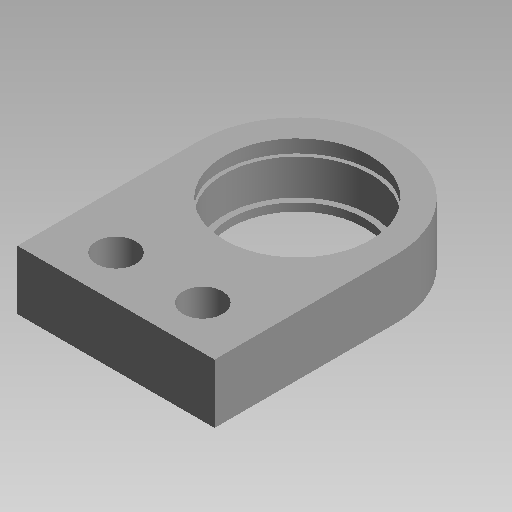
# Autodesk Inventor part: SBGSMA6904ZZ-35_h
Saved by Autodesk Inventor 2021.2 (Build 252289000, 289)
## iProperties
Part Number: SBGSMA6904ZZ-35_h
Material: 一般
Catalog Web Link: www.cadenas.de
Description: BGSMA, BGSMAB, SBGSMA_housing-Bearing with Housings - Front Installation Type
Vendor: MISUMI
Document SubType Name: Modeling
Designer: partserver
Manufacturer: MISUMI
Mass: 30.8974 g
Surface Area: 106.57 cm^2
Volume: 30.8974 cm^3
Density: 1 g/cm^3
Appearance: PSOLRGB-192-192-192
Category: PARTsolutions
Company: MISUMI
PSOL_IDENT_0: {$CADENAS_DATA\23d-libs\misumi\metric\12_bearing_holders\bgsma\bgsma_housing.prj},219 {VTYP=3D},{NB=
PSOL_IDENT_1: SBGSMA6904ZZ-35_h},{LINA=SBGSMA6904ZZ-35},{NN=BGSMA, BGSMAB, SBGSMA_housing},{DATE=30.03.2018 01:48:
PSOL_IDENT_2: 31},{GEOMDATE=13.07.2015 10:26:00},{VERSION=},{LINEID=100},{WBVAR=MATB,STH,SEAL,HH,ALT1},{WBNUMERIC=
PSOL_IDENT_3: HH}  {NB=SBGSMA6904ZZ-35_h},{LINA=SBGSMA6904ZZ-35},{KT=DUMMY},{PN=SBGSMA6904ZZ-35},{TYPE=SBGSMA},{MA
PSOL_IDENT_4: TB=STS},{MATBALG= 'ST','Steel','STS','Stainless Steel' },{STH=},{STHALG= '','-' },{ARR=304 Stainless
PSOL_IDENT_5: Steel},{ARRALG=-S},{BN=6904},{SEAL=ZZ},{SEALALG= 'ZZ','ZZ(Double Shielded)','VV','VV(Non-contact Ru
PSOL_IDENT_6: bber Seal)','DD','DD(Contact Rubber Seal)' },{HH=35},{HHALG=35,45,55},{DD=20},{D=37},{DDHH=34},{B=9}
PSOL_IDENT_7: ,{H=71.0},{HH1=11},{L=50},{L1=22},{T=15},{DD1=10},{ALT1=},{ALT1ALG= '','Bearing and Retaining Ring A
PSOL_IDENT_8: ssembled','NA','with NA (Bearing and Retaining Ring not Assembled)' },{ALT1PN=},{DD2=39.0},{TT=1.50}
NB: SBGSMA6904ZZ-35_h
NN: BGSMA, BGSMAB, SBGSMA_housing
NT: Bearing with Housings - Front Installation Type
NBSYN: $PN._h
LINA: SBGSMA6904ZZ-35
CATALOG: Misumi
PN: SBGSMA6904ZZ-35
MATB: Stainless Steel
STH: -
ARR: 304 Stainless Steel
BN: 6904
SEAL: ZZ(Double Shielded)
HH: 35
DD: 20
D: 37
DDHH: 34
B: 9
H: 71
HH1: 11
L: 50
L1: 22
T: 15
DD1: 10
ALT1: Bearing and Retaining Ring Assembled
SUPPLIER: MISUMI
ARTICLENO: SBGSMA6904ZZ-35_h
BOMINFO: SBGSMA6904ZZ-35
CREATOR: CADENAS GmbH
d17: 0.000 mm
Title: SBGSMA6904ZZ-35
Author: Cadenas PARTsolutions
Comments: Bearing with Housings - Front Installation Type
Autodesk Inventor part; units mm, degrees
sketch "Sketch_7" plane through (0, 0, 0) normal (0, 0, 1) x (1, 0, 0)
  line L0 (-25, 46) -> (-25, 0)
  line L1 (-25, 0) -> (25, 0)
  line L2 (25, 0) -> (25, 46)
  arc A0 (25, 46) -> (-25, 46) centre (0, 46) ccw
  constraints: 6 end point, 2 point on circle, 1 centre point
extrude "Extrusion1" add sketch "Sketch_7" against normal blind 15
sketch "Sketch_8" plane through (0, 0, 0) normal (1, 0, 0) x (0, 0, -1)
  line L0 (15, 46) -> (2, 46)
  line L1 (2, 46) -> (2, 64.5)
  line L2 (2, 64.5) -> (11, 64.5)
  line L3 (11, 64.5) -> (11, 65.5)
  line L4 (11, 65.5) -> (12.5, 65.5)
  line L5 (12.5, 65.5) -> (12.5, 64.5)
  line L6 (12.5, 64.5) -> (15, 64.5)
  line L7 (15, 64.5) -> (15, 46)
  line L8 (15, 46) -> (2, 46)
  constraints: 18 end point
revolve "Revolution1" cut sketch "Sketch_8" angle 360 about axis through (0, 46, -15) along (0, 0, -1)
sketch "Sketch_1" plane through (0, 0, 0) normal (1, 0, 0) x (0, 0, -1)
  line L0 (15, 46) -> (0, 46)
  line L1 (0, 46) -> (0, 63)
  line L2 (0, 63) -> (15, 63)
  line L3 (15, 63) -> (15, 46)
  line L4 (15, 46) -> (0, 46)
  constraints: 10 end point
revolve "Revolution2" cut sketch "Sketch_1" angle 360 about axis through (0, 46, -15) along (0, 0, -1)
sketch "Sketch4" plane through (0, 0, -15) normal (0, 0, -1) x (-1, 0, 0)
  point P0 (11, 11)
hole "Hole1" at (-11, 11, -15) direction (0, 0, 1) diameter 10 depth 15
pattern_linear "Rectangular Pattern1" count 2 spacing 22 along (1, 0, 0) of "Hole1"
ref_plane "to_bearing_XY" through (0, 46, -6.5) normal (0, 0, 1) x (1, 0, 0)
ref_plane "to_bearing_YZ" through (0, 46, -6.5) normal (1, 0, 0) x (0, 1, 0)
ref_plane "to_bearing_ZX" through (0, 46, -6.5) normal (0, 1, 0) x (0, 0, 1)
ref_plane "to_retaining_ring_XY" through (0, 46, -12.5) normal (0, 0, -1) x (1, 0, 0)
ref_plane "to_retaining_ring_YZ" through (0, 46, -12.5) normal (1, 0, 0) x (0, -1, 0)
ref_plane "to_retaining_ring_ZX" through (0, 46, -12.5) normal (0, -1, 0) x (0, 0, -1)
body "Solid1"
